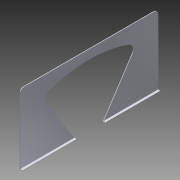
# Autodesk Inventor part: Fin_holed
Saved by Autodesk Inventor 2015 (Build 190159000, 159)
## iProperties
Created: 2015-08-21
Part Number: Fin_holed
Material: Aluminum 6061
Document SubType Name: Modeling
Designer: Kyle
Density: 2.7 g/cm^3
Appearance: Aluminum - Flat
Author: Kyle
Autodesk Inventor part; units mm, degrees
ref_plane "YZ Plane" through (0, 0, 0) normal (1, 0, 0) x (0, 1, 0)
ref_plane "XZ Plane" through (0, 0, 0) normal (0, 1, 0) x (-1, 0, 0)
ref_plane "XY Plane" through (0, 0, 0) normal (0, 0, 1) x (1, 0, 0)
sketch "Sketch1" plane through (0, 0, 0) normal (0, 0, 1) x (1, 0, 0)
  line L0 (0, 0) -> (1.8311, 0)
  line L1 (0, 0) -> (0, 45.085)
  line L2 (0.381, 45.085) -> (0.381, 0.381)
  line L3 (0.381, 0.381) -> (1.8311, 0.381)
  line L4 (1.8311, 0.381) -> (1.8311, 0)
  line L5 (0.381, 45.085) -> (0, 45.085)
  dimension "d0" = 1.8311
  dimension "d1" = 45.085
  dimension "d2" = 0.381
  constraints: 12 end point, 2 vertical, 1 horizontal, 1 perpendicular, 1 other
  measures "d0" distance of L0.start L0.end
  measures "d1" distance of L0.start L1.end
  measures "d2" distance between parallel lines of L1 L2
extrude "Extrusion1" add sketch "Sketch1" along normal blind 88.9
fillet "Fillet1" radius 2.54 2 edges at (0.1905, 45.085, 88.9) (0.1905, 45.085, 0)
sketch "Sketch2" plane through (0, 0, 0) normal (-1, 0, 0) x (0, 0, 1)
  line L0 (0, 0) -> (88.9, 0) projected
  circle A0 centre (40.005, 0) radius 3.175
  circle A1 centre (48.895, 0) radius 3.2307
  dimension "d6" = 6.35
  dimension "d7" = 8.89
  dimension "d8" = 40.005
  constraints: 2 centre point, 2 point on line
  measures "d6" diameter of A0
  measures "d7" distance of A0.centre A1.centre
  measures "d8" distance of L0.end A1.centre
extrude "Extrusion2" cut sketch "Sketch2" against normal blind 88.9
sketch "Sketch3" plane through (0, 0, 0) normal (-1, 0, 0) x (0, 0, 1)
  circle A0 centre (20.32, 31.115) radius 3.4925
  circle A1 centre (68.58, 31.115) radius 3.4925
  line L0 (88.9, 42.545) -> (88.9, 0) projected
  line L1 (0, 42.545) -> (0, 0) projected
  line L2 (2.54, 45.085) -> (86.36, 45.085) projected
  dimension "d11" = 6.985
  dimension "d12" = 6.985
  dimension "d13" = 20.32
  dimension "d14" = 20.32
  dimension "d15" = 13.97
  dimension "d16" = 13.97
  constraints: 2 centre point
  measures "d11" diameter of A0
  measures "d12" diameter of A1
  measures "d13" distance from line of L0 A1.centre
  measures "d14" distance from line of L1 A0.centre
  measures "d15" distance from line of L2 A0.centre
  measures "d16" distance from line of L2 A1.centre
extrude "Extrusion3" cut sketch "Sketch3" against normal blind 88.9
sketch "Sketch4" plane through (0, 0, 0) normal (-1, 0, 0) x (0, 0, 1)
  line L0 (88.9, 42.545) -> (88.9, 0) projected
  line L1 (0, 42.545) -> (0, 0) projected
  line L2 (2.54, 45.085) -> (86.36, 45.085) projected
  line L3 (53.6575, 0) -> (72.39, 28.575)
  line L4 (35.2425, 0) -> (16.51, 28.575)
  arc A0 (69.85, 34.925) -> (19.05, 34.925) centre (44.45, -37.6219) ccw
  arc A1 (19.05, 34.925) -> (16.51, 28.575) centre (20.5495, 30.6422) ccw
  arc A2 (72.39, 28.575) -> (69.85, 34.925) centre (68.3505, 30.6422) ccw
  line L5 (35.2425, 0) -> (53.6575, 0)
  line L6 (52.1257, 0) -> (88.9, 0) projected
  point P0 (44.45, 39.243)
  dimension "d19" = 35.2425
  dimension "d20" = 35.2425
  dimension "d21" = 16.51
  dimension "d22" = 16.51
  dimension "d23" = 16.51
  dimension "d24" = 16.51
  dimension "d25" = 19.05
  dimension "d26" = 19.05
  dimension "d27" = 10.16
  dimension "d28" = 10.16
  dimension "d29" = 5.842
  constraints: 7 point on circle, 6 end point, 3 centre point, 2 tangent, 1 collinear
  measures "d19" distance of L1.end L4.start
  measures "d20" distance from line of L0 L3.start
  measures "d21" distance from line of L1 L4.end
  measures "d22" distance from line of L0 L3.end
  measures "d23" distance from line of L3.end L2
  measures "d24" distance from line of L2 L4.end
  measures "d25" distance from line of L0 A0.start
  measures "d26" distance from line of L1 A0.end
  measures "d27" distance from line of L2 A0.start
  measures "d28" distance from line of L2 A0.end
  measures "d29" distance from line of L2 point (44.45, 39.243)
extrude "Extrusion4" cut sketch "Sketch4" against normal blind 25.4
body "Solid1"
